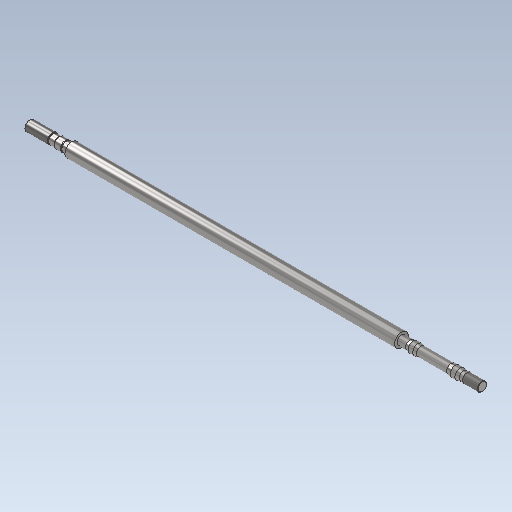
# Autodesk Inventor part: Шток_CPY
Saved by Autodesk Inventor 2021 (Build 250183000, 183)
## iProperties
Created: 2020-11-22
Part Number: Шток_CPY
Material: Сталь, углеродистая
Document SubType Name: Modeling
Designer: Тимоха
Mass: 25235.9 g
Surface Area: 2325.72 cm^2
Volume: 3214.77 cm^3
Density: 7.85 g/cm^3
Appearance: С умеренной полировкой
Author: Тимоха
Autodesk Inventor part; units mm, degrees
ref_plane "YZ Plane" through (0, 0, 0) normal (1, 0, 0) x (0, 1, 0)
ref_plane "XZ Plane" through (0, 0, 0) normal (0, 1, 0) x (-1, 0, 0)
ref_plane "XY Plane" through (0, 0, 0) normal (0, 0, 1) x (1, 0, 0)
sketch "Эскиз1" plane through (0, 0, 0) normal (0, 0, 1) x (1, 0, 0)
  line L0 (0, 0) -> (345, 0)
  line L1 (345, 0) -> (345, 20)
  line L2 (345, 20) -> (280, 20)
  line L3 (0, 0) -> (0, 22.5)
  line L4 (0, 22.5) -> (50, 22.5)
  line L5 (50, 22.5) -> (70, 22.5)
  line L6 (250, 22.5) -> (230, 22.5)
  line L7 (250, 22.5) -> (265, 18.9255)
  line L8 (265, 18.9255) -> (280, 20)
  line L9 (82.7171, 19.4628) -> (70, 22.5)
  line L10 (50, 22.5) -> (36.6597, 19.4628)
  line L11 (36.6597, 19.4628) -> (0, 19.4628)
  line L12 (230, 22.5) -> (211.3782, 19.4628)
  line L13 (211.3782, 19.4628) -> (82.7171, 19.4628)
  dimension "d0" = 345
  dimension "d1" = 20
  dimension "d2" = 65
  dimension "d5" = 22.5
  dimension "d6" = 50
  dimension "d7" = 20
  dimension "d8" = 20
  dimension "d15" = 30
  constraints: 28 end point, 3 horizontal, 3 perpendicular, 2 point on line, 1 vertical
  measures "d0" distance of L0.start L0.end
  measures "d1" distance of L0.end L1.end
  measures "d2" distance of L1.end L2.end
  measures "d5" distance of L0.start L3.end
  measures "d6" distance of L3.end L4.end
  measures "d7" distance of L4.end L5.end
  measures "d8" distance of L6.start L6.end
  measures "d15" horizontal distance of L2.end L6.start
revolve "Вращение1" add sketch "Эскиз1" angle 360 about axis through (0, 0, 0) along (1, 0, 0) contours L3 L11 L10 L5 L9 L13 L12 L6 L7 L8 L2 L1 L0
thread "Резьба1" size "M40x3" class "6g" standard "ANSI Metric M Profile" full length
sketch "Эскиз2" plane through (0, 0, 0) normal (-1, 0, 0) x (0, 0, 1)
  circle A0 centre (0, 0) radius 30
  dimension "d12" = 60
  constraints: 1 centre point, 1 coincident
  measures "d12" diameter of A0
extrude "Выдавливание1" add sketch "Эскиз2" along normal blind 1408
sketch "Эскиз3" plane through (-1408, 0, 0) normal (-1, 0, 0) x (0, 0, 1)
  circle A0 centre (0, 0) radius 22.5
  dimension "d16" = 45
  constraints: 1 centre point, 1 coincident
  measures "d16" diameter of A0
extrude "Выдавливание2" add sketch "Эскиз3" along normal blind 180
sketch "Эскиз4" plane through (0, 0, 0) normal (0, 0, 1) x (1, 0, 0)
  line L0 (-1408, 30) -> (-1408, -30) projected
  line L1 (-1588, 22.5) -> (-1588, -22.5) projected
  line L2 (-1408, -22.5) -> (-1408, 22.5) projected
  line L3 (-1408, 22.5) -> (-1588, 22.5) projected
  line L4 (-1588, 22.5) -> (-1588, -22.5) projected
  line L5 (-1656, 0) -> (-1640, 0)
  line L6 (-1541, 22.5) -> (-1633, 22.5)
  line L7 (-1408, 22.5) -> (-1588, 22.5) projected
  line L8 (-1408, 0) -> (-1408, 20)
  line L9 (-1408, 20) -> (-1432, 20)
  line L10 (-1432, 20) -> (-1434.5, 22.5)
  line L11 (-1408, 22.5) -> (-1588, 22.5) projected
  line L12 (-1434.5, 22.5) -> (-1460.5, 22.5)
  line L13 (-1408, 22.5) -> (-1588, 22.5) projected
  line L14 (-1460.5, 22.5) -> (-1463, 20)
  line L15 (-1463, 20) -> (-1488, 20)
  line L16 (-1488, 20) -> (-1490.5, 22.5)
  line L17 (-1408, 22.5) -> (-1588, 22.5) projected
  line L18 (-1408, 22.5) -> (-1408, 20)
  line L19 (-1490.5, 22.5) -> (-1408, 22.5)
  dimension "d26" = 135
  dimension "d27" = 26
  constraints: 22 end point, 5 point on line, 3 horizontal, 2 perpendicular, 1 collinear, 1 midpoint, 6 other
  measures "d26" angle of L9 L10
  measures "d27" distance of L10.end L12.end
revolve "Вращение2" cut sketch "Эскиз4" angle 360 about axis through (-1656, 0, 0) along (1, 0, 0)
chamfer "Фаска1" distance 2 angle 45 1 edges at (-1588, 0, -22.5)
fillet "Сопряжение1" radius 2 3 edges at (-1488, -20, 0) (-1463, -20, 0) (-1432, -20, 0)
thread "Резьба2" size "M45x4.5" class "6g" standard "ANSI Metric M Profile" full length
chamfer "Фаска2" distance 2 angle 45 1 edges at (345, -20, 0)
